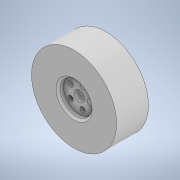
# Autodesk Inventor part: wheel
Saved by Autodesk Inventor 2021 (Build 250183000, 183)
## iProperties
Created: 2021-07-04
Part Number: wheel
Material: Generic
Document SubType Name: Modeling
Designer: Admin
Density: 1 g/cm^3
Appearance: Default
Author: Admin
Autodesk Inventor part; units mm, degrees
ref_plane "YZ Plane" through (0, 0, 0) normal (1, 0, 0) x (0, 1, 0)
ref_plane "XZ Plane" through (0, 0, 0) normal (0, 1, 0) x (-1, 0, 0)
ref_plane "XY Plane" through (0, 0, 0) normal (0, 0, 1) x (1, 0, 0)
sketch "Sketch28" plane through (0, 0, 0) normal (0, 0, 1) x (1, 0, 0)
  point P0 (0, 0)
sketch "Sketch29" plane through (0, 0, 0) normal (0, 0, 1) x (1, 0, 0)
  circle A0 centre (0, 0) radius 40
  dimension "d84" = 80
  constraints: 1 centre point, 1 coincident
  measures "d84" diameter of A0
extrude "Extrusion25" add sketch "Sketch29" along normal blind 30
sketch "Sketch30" plane through (0, 0, 30) normal (0, 0, 1) x (1, 0, 0)
  circle A0 centre (0, 0) radius 15
  dimension "d87" = 30
  constraints: 1 centre point, 1 coincident
  measures "d87" diameter of A0
extrude "Extrusion26" cut sketch "Sketch30" against normal blind 5
sketch "Sketch31" plane through (0, 0, 0) normal (0, 0, -1) x (-1, 0, 0)
  circle A0 centre (0, 0) radius 15
  dimension "d90" = 30
  constraints: 1 centre point, 1 coincident
  measures "d90" diameter of A0
extrude "Extrusion27" cut sketch "Sketch31" against normal blind 5
sketch "Sketch32" plane through (0, 0, 25) normal (0, 0, 1) x (1, 0, 0)
  circle A0 centre (0, 0) radius 5
  dimension "d93" = 10
  constraints: 1 centre point, 1 coincident
  measures "d93" diameter of A0
extrude "Extrusion28" cut sketch "Sketch32" against normal blind 20
sketch "Sketch33" plane through (0, 0, 25) normal (0, 0, 1) x (1, 0, 0)
  circle A0 centre (10, 0) radius 2.5
  circle A1 centre (3.0902, 9.5106) radius 2.5
  circle A2 centre (-8.0902, 5.8779) radius 2.5
  circle A3 centre (-8.0902, -5.8779) radius 2.5
  circle A4 centre (3.0902, -9.5106) radius 2.5
  point P0 (0, 0)
  dimension "d96" = 5
  dimension "d99" = 360
  constraints: 5 centre point, 11 other
  measures "d96" diameter of A0
extrude "Extrusion29" cut sketch "Sketch33" against normal blind 20
chamfer "Chamfer1" distance 2 angle 45 2 edges at (15, 0, 0) (-15, 0, 30)
body "Solid7"
